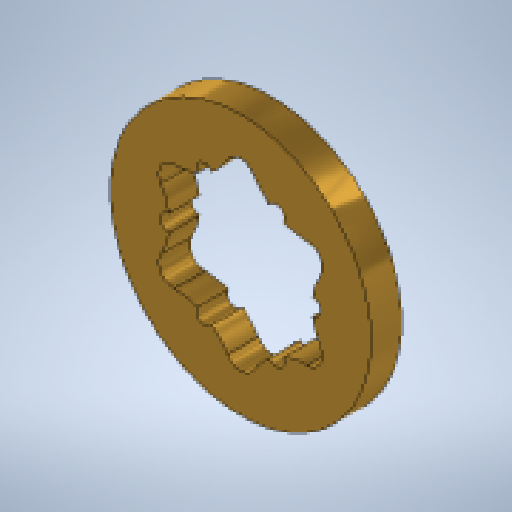
# Autodesk Inventor part: Brass Gryo
Saved by Autodesk Inventor 2023.2 (Build 272271000, 271)
## iProperties
Created: 2023-06-11
Part Number: Brass Gryo
Material: Brass, Soft Yellow
Document SubType Name: Modeling
Designer: Nathan Cai
Density: 8.47 g/cm^3
Appearance: Brass - Satin
Mass: 74.9679 g
Surface Area: 46.9143 cm^2
Volume: 8.85099 cm^3
Author: Nathan Cai
Autodesk Inventor part; units mm, degrees
ref_plane "YZ Plane" through (0, 0, 0) normal (1, 0, 0) x (0, 1, 0)
ref_plane "XZ Plane" through (0, 0, 0) normal (0, 1, 0) x (-1, 0, 0)
ref_plane "XY Plane" through (0, 0, 0) normal (0, 0, 1) x (1, 0, 0)
sketch "Sketch1" plane through (0, 0, 0) normal (0, 0, 1) x (1, 0, 0)
  circle A0 centre (0, 0) radius 26.9875
  circle A1 centre (0, 0) radius 7.9375 construction
  circle A2 centre (0, 0) radius 19.05
  line L0 (0, 0) -> (0, 26.9875) construction
  circle A3 centre (0, 0) radius 3.175 construction
  circle A4 centre (0, 15.875) radius 3.175
  line L1 (0, 15.875) -> (13.7482, 7.9375) construction
  line L2 (13.7482, 7.9375) -> (13.7482, -7.9375) construction
  line L3 (13.7482, -7.9375) -> (0, -15.875) construction
  line L4 (0, -15.875) -> (-13.7482, -7.9375) construction
  line L5 (-13.7482, -7.9375) -> (-13.7482, 7.9375) construction
  line L6 (-13.7482, 7.9375) -> (0, 15.875) construction
  circle A5 centre (13.7482, 7.9375) radius 3.175
  arc A6 (2.7496, 17.4625) -> (13.7482, 11.1125) centre (13.7482, 23.8125) ccw
  arc A7 (-13.7482, 11.1125) -> (-2.7496, 17.4625) centre (-13.7482, 23.8125) ccw
  circle A8 centre (0, 15.875) radius 3.175
  arc A9 (-16.4978, -6.35) -> (-16.4978, 6.35) centre (-27.4963, 0) ccw
  circle A10 centre (-13.7482, 7.9375) radius 3.175
  arc A11 (-2.7496, -17.4625) -> (-13.7482, -11.1125) centre (-13.7482, -23.8125) ccw
  circle A12 centre (-13.7482, -7.9375) radius 3.175
  arc A13 (13.7482, -11.1125) -> (2.7496, -17.4625) centre (13.7482, -23.8125) ccw
  circle A14 centre (0, -15.875) radius 3.175
  arc A15 (16.4978, 6.35) -> (16.4978, -6.35) centre (27.4963, 0) ccw
  circle A16 centre (13.7482, -7.9375) radius 3.175
  circle A17 centre (7.3982, -12.814) radius 1.7526
  circle A18 centre (14.7963, 0) radius 1.7526
  circle A19 centre (7.3982, 12.814) radius 1.7526
  circle A20 centre (-7.3982, 12.814) radius 1.7526
  circle A21 centre (-14.7963, 0) radius 1.7526
  circle A22 centre (-7.3982, -12.814) radius 1.7526
  point P0 (13.7482, -11.1125)
  point P1 (-2.7496, -17.4625)
  point P2 (-16.4978, -6.35)
  point P3 (-13.7482, 11.1125)
  point P4 (-2.7496, 17.4625)
  point P5 (14.9172, 1.7484)
  point P6 (14.9172, -1.7484)
  point P7 (8.9728, -12.0445)
  point P8 (5.9444, -13.7929)
  point P9 (-5.9444, -13.7929)
  point P10 (-8.9728, -12.0445)
  point P11 (-14.9172, -1.7484)
  point P12 (-14.9172, 1.7484)
  point P13 (-8.9728, 12.0445)
  point P14 (-5.9444, 13.7929)
  point P15 (5.9444, 13.7929)
  point P16 (8.9728, 12.0445)
  dimension "d0" = 53.975
  dimension "d13" = 6.35
  dimension "d14" = 6.35
  dimension "d1" = 15.875
  dimension "d4" = 6.35
  dimension "d15" = 12.7
  dimension "d18" = 360
  dimension "d20" = 3.5052
  dimension "d23" = 360
  dimension "d25" = 38.1
  constraints: 15 centre point, 14 end point, 13 point on circle, 6 coincident, 1 point on line, 1 vertical, 1 vertical alignment, 89 other
  measures "d1" diameter of A1
  measures "d4" diameter of A3
  measures "d15" radius of A6
  measures "d20" diameter of A17
  measures "d25" diameter of A2
extrude "Extrusion1" add sketch "Sketch1" along normal blind 6.35 contours A0 | A2 A16 A15 A18 A5 | A5 A6 A19 A4 A2 | A2 A14 A13 A17 A16 | A4 A7 A20 A10 A2 | A2 A12 A11 A22 A14 | A10 A9 A21 A12 A2
body "Solid1"
